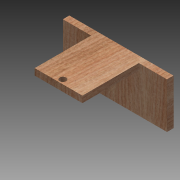
# Autodesk Inventor part: Puller1
Saved by Autodesk Inventor 2014 SP1 (Build 180222100, 222)
## iProperties
Created: 2014-11-12
Part Number: Puller1
Material: Generic
Document SubType Name: Modeling
Designer: AlecShufelt
Density: 1 g/cm^3
Appearance: Default
Author: AlecShufelt
Autodesk Inventor part; units mm, degrees
ref_plane "YZ Plane" through (0, 0, 0) normal (1, 0, 0) x (0, 1, 0)
ref_plane "XZ Plane" through (0, 0, 0) normal (0, 1, 0) x (-1, 0, 0)
ref_plane "XY Plane" through (0, 0, 0) normal (0, 0, 1) x (1, 0, 0)
sketch "Sketch1" plane through (0, 0, 0) normal (0, 0, 1) x (1, 0, 0)
  line L0 (0, 0) -> (304.8, 0)
  line L1 (304.8, 0) -> (304.8, 133.35)
  line L2 (304.8, 133.35) -> (0, 133.35)
  line L3 (0, 133.35) -> (0, 0)
  dimension "d0" = 304.8
  dimension "d1" = 133.35
  constraints: 8 end point, 2 parallel, 1 horizontal, 1 perpendicular
  measures "d0" distance of L2.end L1.end
  measures "d1" distance of L1.end L0.end
extrude "Extrusion1" add sketch "Sketch1" along normal blind 19.05
sketch "Sketch2" plane through (0, 0, 19.05) normal (0, 0, 1) x (1, 0, 0)
  line L0 (304.8, 133.35) -> (0, 133.35) projected
  line L1 (0, 133.35) -> (0, 0) projected
  line L2 (82.55, 133.35) -> (222.25, 133.35)
  line L3 (222.25, 133.35) -> (222.25, 114.3)
  line L4 (222.25, 114.3) -> (82.55, 114.3)
  line L5 (82.55, 114.3) -> (82.55, 133.35)
  dimension "d4" = 139.7
  dimension "d5" = 19.05
  dimension "d6" = 82.55
  constraints: 8 end point, 2 parallel, 1 horizontal, 1 perpendicular, 1 point on line
  measures "d4" distance of L3.end L4.end
  measures "d5" distance of L2.end L3.end
  measures "d6" distance between parallel lines of L1 L5
extrude "Extrusion2" add sketch "Sketch2" along normal blind 165.1
sketch "Sketch3" plane through (82.55, 114.3, 19.05) normal (0, -1, 0) x (1, 0, 0)
  line L0 (0, 165.1) -> (139.7, 165.1) projected
  circle A0 centre (69.85, 152.4) radius 9.525
  point P0 (-82.55, -19.05)
  dimension "d9" = 19.05
  dimension "d10" = 12.7
  constraints: 1 centre point
  measures "d9" diameter of A0
  measures "d10" distance from line of L0 A0.centre
extrude "Extrusion3" cut sketch "Sketch3" against normal blind 165.1
body "Solid1"
